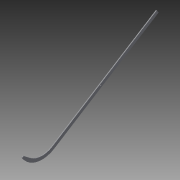
# Autodesk Inventor part: MammothTusk
Saved by Autodesk Inventor 2013 (Build 170138000, 138)
## iProperties
Created: 2014-01-11
Part Number: MammothTusk
Material: Generic
Document SubType Name: Modeling
Designer: 215152
Density: 1 g/cm^3
Author: 215152
Autodesk Inventor part; units mm, degrees
ref_plane "YZ Plane" through (0, 0, 0) normal (1, 0, 0) x (0, 1, 0)
ref_plane "XZ Plane" through (0, 0, 0) normal (0, 1, 0) x (-1, 0, 0)
ref_plane "XY Plane" through (0, 0, 0) normal (0, 0, 1) x (1, 0, 0)
sketch "Sketch1" plane through (0, 0, 0) normal (1, 0, 0) x (0, 1, 0)
  circle A0 centre (0, 0) radius 152.4
  line L0 (-76.2507, 131.953) -> (76.2507, 131.953)
  line L1 (76.2507, 131.953) -> (76.2507, -131.953)
  line L2 (76.2507, -131.953) -> (-76.2507, -131.953)
  line L3 (-76.2507, -131.953) -> (-76.2507, 131.953)
  line L4 (-76.2507, 131.953) -> (76.2507, -131.953) construction
  line L5 (76.2507, 131.953) -> (-76.2507, -131.953) construction
  line L6 (-76.2507, 131.953) -> (-88.9591, 153.9452)
  line L7 (-76.2507, -131.953) -> (-88.9591, -153.9452)
  arc A1 (-88.9591, 153.9452) -> (-88.9591, -153.9452) centre (0, 0) ccw
  line L8 (-88.9591, 153.9452) -> (-177.8, 153.9452)
  line L9 (-177.8, 153.9452) -> (-177.8, -354.0548)
  line L10 (-177.8, -354.0548) -> (0, -354.0548)
  line L11 (0, -354.0548) -> (0, -430.2548)
  line L12 (0, -430.2548) -> (-127, -430.2548)
  line L13 (-127, -430.2548) -> (-127, -354.0548)
  line L14 (-127, -430.2548) -> (-177.8, -430.2548)
  line L15 (-177.8, -430.2548) -> (-177.8, -354.0548)
  line L16 (0, -354.0548) -> (12.7, -354.0548)
  line L17 (12.7, -354.0548) -> (-150.4905, -94.6861)
  line L18 (12.7, -354.0548) -> (34.1986, -340.5282)
  line L19 (34.1986, -340.5282) -> (-128.9918, -81.1595)
  line L20 (12.7, -354.0548) -> (60.6438, -430.2548)
  line L21 (60.6438, -430.2548) -> (82.1424, -416.7282)
  line L22 (82.1424, -416.7282) -> (34.1986, -340.5282)
  line L23 (-177.8, 0) -> (127, 0)
  circle A2 centre (127, 0) radius 304.8
  line L24 (-82.6049, 142.9491) -> (-121.1364, 92.4756)
  line L25 (0, -430.2548) -> (0, -455.6548)
  line L26 (0, -455.6548) -> (235.9429, -455.6548)
  line L27 (82.1424, -416.7282) -> (106.6344, -455.6548)
  line L28 (106.6344, -455.6548) -> (85.1357, -469.1814)
  line L29 (85.1357, -469.1814) -> (60.6438, -430.2548)
  line L30 (95.885, -462.4181) -> (91.6297, -455.6548)
  line L31 (91.6297, -455.6548) -> (98.393, -466.4042)
  line L32 (98.393, -466.4042) -> (120.7006, -452.3686)
  line L33 (106.6344, -455.6548) -> (109.1423, -459.6409)
  line L34 (98.393, -466.4042) -> (67.8539, -485.6188)
  line L35 (85.1357, -469.1814) -> (87.6437, -473.1674)
  line L36 (109.1423, -459.6409) -> (87.6437, -473.1674)
  arc A3 (-88.9591, 153.9452) -> (-150.4905, -94.6861) centre (0, 0) ccw
  line L37 (-128.9918, -81.1595) -> (109.1423, -459.6409)
  line L38 (-150.4905, -94.6861) -> (87.6437, -473.1674)
  line L39 (87.6437, -473.1674) -> (109.1423, -459.6409)
  dimension "d5" = 304.8
  dimension "d6" = 263.906
  dimension "d7" = 25.4
  dimension "d8" = 25.4
  dimension "d9" = 508
  dimension "d10" = 76.2
  dimension "d11" = 127
  dimension "d12" = 12.7
  dimension "d13" = 25.4
  dimension "d14" = 25.4
  dimension "d15" = 304.8
  dimension "d16" = 25.4
  dimension "d17" = 12.7
  constraints: 80 end point, 18 perpendicular, 9 point on circle, 8 collinear, 8 parallel, 8 tangent, 6 point on line, 4 midpoint, 3 centre point, 2 coincident, 1 horizontal, 1 horizontal alignment, 2 other
  measures "d5" diameter of A0
  measures "d6" distance of L0.end L1.end
  measures "d7" distance of L0.start L6.end
  measures "d8" distance of L2.end L7.end
  measures "d9" distance of L8.end L9.end
  measures "d10" distance of L10.end L11.end
  measures "d11" distance of L11.end L12.end
  measures "d12" distance of L10.end L16.end
  measures "d13" distance of L16.end L18.end
  measures "d14" distance of L20.end L21.end
  measures "d15" distance of L23.start L23.end
  measures "d16" distance of L11.end L25.end
  measures "d17" distance of L30.end L31.end
extrude "Extrusion1" add sketch "Sketch1" along normal blind 6.35 contours A0 L23 A1 L6 L24 | L19 L7 A1 L23 A0 | L19 A2 L17 A1 L7 | L19 L18 L17 A2 | L22 L21 L20 L18 | L27 L26 L29 L21 | L28 L30 L26 | L33 L32 L31 L28 | L26 L30 L28 L29 | L31 L34 L35 L28
sketch "Sketch2" plane through (6.35, 0, 0) normal (1, 0, 0) x (0, 0, -1)
  line L0 (473.1674, 87.6437) -> (459.6409, 109.1423) projected
  line L1 (-142.9491, -82.6049) -> (-153.9452, -88.9591) projected
  line L2 (466.4042, 98.393) -> (455.4081, 92.0388)
  circle A0 centre (455.4081, 92.0388) radius 3.175
  dimension "d20" = 12.7
  dimension "d21" = 6.35
  constraints: 2 end point, 1 centre point, 1 coincident, 1 midpoint, 1 parallel
  measures "d20" distance of L2.start L2.end
  measures "d21" diameter of A0
extrude "Extrusion2" cut sketch "Sketch2" against normal blind 25.4
sketch "Sketch3" plane through (6.35, 109.1423, -459.6409) normal (0, 0.5325427, -0.8464031) x (-1, 0, 0)
  line L0 (6.35, -25.4) -> (6.35, 0) projected
  line L1 (6.35, 0) -> (0, 0) projected
  line L2 (0, -25.4) -> (0, 0) projected
  line L3 (6.35, -25.4) -> (0, -25.4) projected
  point P0 (6.35, 152.4)
extrude "Extrusion3" add sketch "Sketch3" along normal blind 508
body "Solid1"
